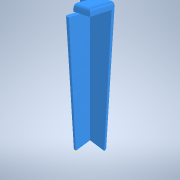
# Autodesk Inventor part: DoosjeHoeken
Saved by Autodesk Inventor 2021 (Build 250183000, 183)
## iProperties
Created: 2021-03-11
Part Number: DoosjeHoeken
Material: ABS Plastic
Document SubType Name: Modeling
Designer: ZiweZhang
Density: 1.06 g/cm^3
Appearance: Cyan
Author: ZiweZhang
Autodesk Inventor part; units mm, degrees
ref_plane "YZ Plane" through (0, 0, 0) normal (1, 0, 0) x (0, 1, 0)
ref_plane "XZ Plane" through (0, 0, 0) normal (0, 1, 0) x (-1, 0, 0)
ref_plane "XY Plane" through (0, 0, 0) normal (0, 0, 1) x (1, 0, 0)
sketch "Sketch1" plane through (0, 0, 0) normal (0, 1, 0) x (-1, 0, 0)
  line L0 (15, 0) -> (15, -15)
  line L1 (15, -15) -> (0, -15)
  line L2 (0, -15) -> (0, -12)
  line L3 (0, -12) -> (12, -12)
  line L4 (12, -12) -> (12, 0)
  line L5 (12, 0) -> (15, 0)
  point P0 (0, 0)
  dimension "d0" = 15
  dimension "d1" = 15
  dimension "d10" = 3
  dimension "d11" = 12
  dimension "d12" = 12
  constraints: 12 end point, 1 horizontal, 1 perpendicular
  measures "d0" distance of L0.end L1.end
  measures "d1" distance of L0.start L0.end
  measures "d10" distance of L1.end L2.end
  measures "d11" distance of L2.end L3.end
  measures "d12" distance of L3.end L4.end
extrude "Extrusion1" add sketch "Sketch1" along normal blind 86
sketch "Sketch4" plane through (-12, 0, 0) normal (1, 0, 0) x (0, 0, -1)
  line L0 (0, 0) -> (0, 86) projected
  line L1 (12, 0) -> (12, 86) projected
  line L2 (0, 86) -> (12, 86)
  line L3 (12, 86) -> (12, 83)
  line L4 (12, 83) -> (0, 83)
  line L5 (0, 83) -> (0, 86)
  dimension "d13" = 3
  constraints: 8 end point, 2 parallel, 1 horizontal, 1 perpendicular, 1 point on line
  measures "d13" distance of L2.end L3.end
extrude "Extrusion3" add sketch "Sketch4" along normal blind 3
sketch "Sketch6" plane through (-12, 0, -12) normal (0, 0, 1) x (1, 0, 0)
  line L0 (3, 86) -> (12, 86) projected
  line L1 (12, 86) -> (3, 86)
  line L2 (3, 86) -> (3, 83)
  line L3 (3, 83) -> (12, 83)
  line L4 (12, 83) -> (12, 86)
  point P0 (12, 0)
  constraints: 8 end point, 2 parallel, 1 horizontal, 1 perpendicular
extrude "Extrusion4" add sketch "Sketch6" along normal blind 12
fillet "Fillet3" radius 2 7 edges at (-7.5, 86, -15) (-15, 86, -7.5) (-15, 43, -15) (0, 43, -15) (-7.5, 86, 0) (0, 86, -7.5) (-15, 43, 0)
sketch "Sketch11" plane through (0, 86, 0) normal (0, 1, 0) x (1, 0, 0)
  arc A0 (-15, 2) -> (-13, 0) centre (-13, 2) ccw projected
  line L0 (-13, 0) -> (-10, 0)
  line L1 (-15, 9) -> (-15, 0)
  line L2 (-15, 0) -> (-13, 0)
  line L3 (-9, 9) -> (-9, 0)
  line L4 (-9, 0) -> (-15, 0)
  line L5 (-9, 9) -> (-15, 9)
  point P0 (0, 0)
  point P1 (-13, 0)
  constraints: 12 end point, 1 collinear, 1 horizontal, 1 perpendicular
extrude "Extrusion7" cut sketch "Sketch11" against normal blind 6
sketch "Sketch12" plane through (-12, 0, 0) normal (1, 0, 0) x (0, 0, -1)
  line L0 (0, 33) -> (9, 33) construction
  line L1 (0, 0) -> (0, 80) projected
  line L2 (0, 36) -> (9, 36)
  line L3 (0, 39) -> (0, 36)
  line L4 (9, 36) -> (9, 39)
  line L5 (0, 39) -> (9, 39)
  line L6 (0, 0) -> (0, 80) projected
  line L7 (0, 36) -> (0, 39)
  constraints: 12 end point, 2 perpendicular, 1 collinear, 1 horizontal, 1 point on line
extrude "Extrusion8" cut sketch "Sketch12" against normal through all
body "Solid1"
